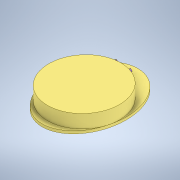
# Autodesk Inventor part: Hat
Saved by Autodesk Inventor 2020.4 (Build 244396000, 396)
## iProperties
Created: 2021-05-01
Part Number: Hat
Material: Generic
Document SubType Name: Modeling
Designer: armin
Density: 1 g/cm^3
Appearance: Default
Author: armin
Autodesk Inventor part; units mm, degrees
note: some values were not read from the file. Chosen so that the rebuilt part matches the saved one: direction of "Emboss1".
ref_plane "YZ Plane" through (0, 0, 0) normal (1, 0, 0) x (0, 1, 0)
ref_plane "XZ Plane" through (0, 0, 0) normal (0, 1, 0) x (-1, 0, 0)
sketch "Sketch1" plane through (0, 0, 0) normal (0, 1, 0) x (-1, 0, 0)
  ellipse E0 centre (0, -4.3604) end of major axis (0, 31.5492) minor radius 27.0568
  ellipse E1 centre (0, -7.8745) end of major axis (0, -12.399) minor radius 3.571
  point P0 (0.4642, 6.4079)
  constraints: 1 centre point, 3 other
extrude "Extrusion1" add sketch "Sketch1" along normal blind 2 contours E0 | E1
sketch "Sketch2" plane through (0, 2, 0) normal (0, 1, 0) x (1, 0, 0)
  ellipse E0 centre (0, 0) end of major axis (0, -27.5508) minor radius 26.511
  ellipse E1 centre (0, 4.3604) end of major axis (0, -31.5492) minor radius 27.0568 projected
  point P0 (8.845, -15.5857)
  point P1 (-8.845, -15.5857)
  constraints: 1 coincident, 3 other
extrude "Extrusion2" add sketch "Sketch2" along normal blind 10 contours E0
ref_plane "Work Plane1" through (0, 0, -57) normal (0, 0, 1) x (1, 0, 0)
sketch "Sketch3" plane through (0, 0, -57) normal (0, 0, 1) x (1, 0, 0)
  line L0 (0, 7.5145) -> (2.0048, 6.0468)
  line L1 (2.0048, 6.0468) -> (4.6288, 9.6309)
  line L2 (4.6288, 9.6309) -> (6.2039, 8.4777)
  line L3 (6.2039, 8.4777) -> (1.9982, 3.5336)
  line L4 (1.9982, 3.5336) -> (0, 5.2333)
  line L5 (0, 5.2333) -> (-1.4459, 3.5336)
  line L6 (-1.4459, 3.5336) -> (-6.886, 9.626)
  line L7 (-6.886, 9.626) -> (-5.8582, 10.2166)
  line L8 (-5.8582, 10.2166) -> (-1.0292, 6.1088)
  line L9 (-1.0292, 6.1088) -> (0, 7.5145)
  point P0 (0, 0)
  constraints: 20 end point, 5 perpendicular, 2 point on line
emboss "Emboss1" sketch "Sketch3" operation add depth 3 direction (0, 0, 1)
body "Solid1"
